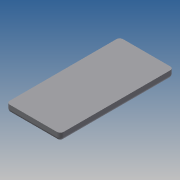
# Autodesk Inventor part: Part2
Saved by Autodesk Inventor 2014 (Build 180170000, 170)
## iProperties
Created: 2014-04-29
Part Number: Part2
Material: Generic
Document SubType Name: Modeling
Designer: 1770749
Density: 1 g/cm^3
Appearance: Default
Author: 1770749
Autodesk Inventor part; units mm, degrees
ref_plane "YZ Plane" through (0, 0, 0) normal (1, 0, 0) x (0, 1, 0)
ref_plane "XZ Plane" through (0, 0, 0) normal (0, 1, 0) x (-1, 0, 0)
ref_plane "XY Plane" through (0, 0, 0) normal (0, 0, 1) x (1, 0, 0)
sketch "Sketch1" plane through (0, 0, 0) normal (0, 0, 1) x (1, 0, 0)
  line L0 (0, 0) -> (59.18, 0)
  line L1 (59.18, 0) -> (59.18, 124.44)
  line L2 (59.18, 124.44) -> (0, 124.44)
  line L3 (0, 124.44) -> (0, 0)
  dimension "d0" = 59.18
  dimension "d1" = 124.44
  constraints: 8 end point, 2 parallel, 1 horizontal, 1 perpendicular
  measures "d0" distance of L2.end L1.end
  measures "d1" distance of L1.end L0.end
extrude "Extrusion1" add sketch "Sketch1" against normal blind 8.5
fillet "Fillet1" radius 3.74 1 edges at (29.59, 124.44, -8.5)
fillet "Fillet2" radius 3.74 1 edges at (29.59, 0, -8.5)
fillet "Fillet3" radius 3.74 5 edges at (59.18, 1.0954, -7.4046) (59.18, 0, -2.38) (59.18, 123.3446, -7.4046) (59.18, 124.44, -2.38) (59.18, 62.22, -8.5)
fillet "Fillet4" radius 3.74 5 edges at (0, 123.3446, -7.4046) (0, 124.44, -2.38) (0, 1.0954, -7.4046) (0, 0, -2.38) (0, 62.22, -8.5)
body "Solid1"
